Autodesk Inventor part; units mm, degrees
(part 4 of 4)
sketch "Sketch8" plane through (0, 0, 5) normal (0, 0, 1) x (1, 0, 0)
  line L0 (14.5144, 16.8863) -> (85.9619, 16.8863) construction
  line L1 (85.9619, 16.8863) -> (85.9619, -28.4978) construction
  line L2 (85.9619, -28.4978) -> (14.5144, -28.4978) construction
  line L3 (14.5144, -28.4978) -> (14.5144, 16.8863) construction
  line L4 (50.2381, 55.1961) -> (50.2381, 17.6773) construction
  line L5 (0, -39.5) -> (0, 79.5) construction
  spline S0 degree 2 poles (33.201, 11.0366) (32.522, 10.6859) (31.5146, 10.6859) knots 0 0 0 1 1 1
  spline S1 degree 2 poles (31.5146, 10.6859) (30.2066, 10.6859) (28.637, 12.3334) (28.637, 13.6748) knots 0 0 0 1 2 2 2
  spline S2 degree 2 poles (28.637, 13.6748) (28.637, 15.1108) (30.407, 16.8863) (31.7595, 16.8863) knots 0 0 0 1 2 2 2
  spline S3 degree 2 poles (31.7595, 16.8863) (32.6277, 16.8863) (33.201, 16.6414) knots 0 0 0 1 1 1
  line L6 (33.201, 16.6414) -> (33.201, 15.6507)
  spline S4 degree 2 poles (33.201, 15.6507) (32.5943, 16.0125) (31.8597, 16.0125) knots 0 0 0 1 1 1
  spline S5 degree 2 poles (31.8597, 16.0125) (30.8856, 16.0125) (29.6778, 14.7657) (29.6778, 13.7249) knots 0 0 0 1 2 2 2
  spline S6 degree 2 poles (29.6778, 13.7249) (29.6778, 12.7286) (30.8077, 11.5542) (31.7261, 11.5542) knots 0 0 0 1 2 2 2
  spline S7 degree 2 poles (31.7261, 11.5542) (32.5776, 11.5542) (33.201, 11.955) knots 0 0 0 1 1 1
  line L7 (33.201, 11.955) -> (33.201, 11.0366)
  line L8 (39.1565, 10.7861) -> (38.1602, 10.7861)
  line L9 (38.1602, 10.7861) -> (38.1602, 13.391)
  line L10 (38.1602, 13.391) -> (35.3327, 13.391)
  line L11 (35.3327, 13.391) -> (35.3327, 10.7861)
  line L12 (35.3327, 10.7861) -> (34.3365, 10.7861)
  line L13 (34.3365, 10.7861) -> (34.3365, 16.7861)
  line L14 (34.3365, 16.7861) -> (35.3327, 16.7861)
  line L15 (35.3327, 16.7861) -> (35.3327, 14.2648)
  line L16 (35.3327, 14.2648) -> (38.1602, 14.2648)
  line L17 (38.1602, 14.2648) -> (38.1602, 16.7861)
  line L18 (38.1602, 16.7861) -> (39.1565, 16.7861)
  line L19 (39.1565, 16.7861) -> (39.1565, 10.7861)
  line L20 (45.5684, 10.7861) -> (44.4775, 10.7861)
  line L21 (44.4775, 10.7861) -> (43.9376, 12.3112)
  line L22 (43.9376, 12.3112) -> (41.5776, 12.3112)
  line L23 (41.5776, 12.3112) -> (41.0545, 10.7861)
  line L24 (41.0545, 10.7861) -> (39.9691, 10.7861)
  line L25 (39.9691, 10.7861) -> (42.2177, 16.7861)
  line L26 (42.2177, 16.7861) -> (43.3365, 16.7861)
  line L27 (43.3365, 16.7861) -> (45.5684, 10.7861)
  line L28 (43.6704, 13.1238) -> (42.8411, 15.5171)
  spline S8 degree 2 poles (42.8411, 15.5171) (42.8021, 15.634) (42.7576, 15.8956) knots 0 0 0 1 1 1
  line L29 (42.7576, 15.8956) -> (42.7409, 15.8956)
  spline S9 degree 2 poles (42.7409, 15.8956) (42.7075, 15.6563) (42.6574, 15.5171) knots 0 0 0 1 1 1
  line L30 (42.6574, 15.5171) -> (41.8337, 13.1238)
  line L31 (41.8337, 13.1238) -> (43.6704, 13.1238)
  line L32 (49.7149, 10.7861) -> (46.3921, 10.7861)
  line L33 (46.3921, 10.7861) -> (46.3921, 16.7861)
  line L34 (46.3921, 16.7861) -> (47.3884, 16.7861)
  line L35 (47.3884, 16.7861) -> (47.3884, 11.6266)
  line L36 (47.3884, 11.6266) -> (49.7149, 11.6266)
  line L37 (49.7149, 11.6266) -> (49.7149, 10.7861)
  line L38 (57.0285, 10.7861) -> (56.0433, 10.7861)
  line L39 (56.0433, 10.7861) -> (56.0433, 14.6711)
  spline S10 degree 2 poles (56.0433, 14.6711) (56.0433, 15.1442) (56.099, 15.8344) knots 0 0 0 1 1 1
  line L40 (56.099, 15.8344) -> (56.0823, 15.8344)
  spline S11 degree 2 poles (56.0823, 15.8344) (55.9932, 15.4448) (55.9209, 15.2722) knots 0 0 0 1 1 1
  line L41 (55.9209, 15.2722) -> (54.1287, 10.7861)
  line L42 (54.1287, 10.7861) -> (53.4441, 10.7861)
  line L43 (53.4441, 10.7861) -> (51.6463, 15.2388)
  spline S12 degree 2 poles (51.6463, 15.2388) (51.5739, 15.4336) (51.4904, 15.8344) knots 0 0 0 1 1 1
  line L44 (51.4904, 15.8344) -> (51.4738, 15.8344)
  spline S13 degree 2 poles (51.4738, 15.8344) (51.5071, 15.4782) (51.5071, 14.66) knots 0 0 0 1 1 1
  line L45 (51.5071, 14.66) -> (51.5071, 10.7861)
  line L46 (51.5071, 10.7861) -> (50.5832, 10.7861)
  line L47 (50.5832, 10.7861) -> (50.5832, 16.7861)
  line L48 (50.5832, 16.7861) -> (51.9858, 16.7861)
  line L49 (51.9858, 16.7861) -> (53.561, 12.7898)
  spline S14 degree 2 poles (53.561, 12.7898) (53.7446, 12.3279) (53.8003, 12.1052) knots 0 0 0 1 1 1
  line L50 (53.8003, 12.1052) -> (53.817, 12.1052)
  spline S15 degree 2 poles (53.817, 12.1052) (53.9728, 12.5783) (54.0674, 12.8065) knots 0 0 0 1 1 1
  line L51 (54.0674, 12.8065) -> (55.676, 16.7861)
  line L52 (55.676, 16.7861) -> (57.0285, 16.7861)
  line L53 (57.0285, 16.7861) -> (57.0285, 10.7861)
  line L54 (61.8708, 10.7861) -> (58.5034, 10.7861)
  line L55 (58.5034, 10.7861) -> (58.5034, 16.7861)
  line L56 (58.5034, 16.7861) -> (61.7372, 16.7861)
  line L57 (61.7372, 16.7861) -> (61.7372, 15.9401)
  line L58 (61.7372, 15.9401) -> (59.4997, 15.9401)
  line L59 (59.4997, 15.9401) -> (59.4997, 14.2425)
  line L60 (59.4997, 14.2425) -> (61.5647, 14.2425)
  line L61 (61.5647, 14.2425) -> (61.5647, 13.4021)
  line L62 (61.5647, 13.4021) -> (59.4997, 13.4021)
  line L63 (59.4997, 13.4021) -> (59.4997, 11.6266)
  line L64 (59.4997, 11.6266) -> (61.8708, 11.6266)
  line L65 (61.8708, 11.6266) -> (61.8708, 10.7861)
  line L66 (67.5758, 10.7861) -> (66.4125, 10.7861)
  line L67 (66.4125, 10.7861) -> (65.4552, 12.3947)
  spline S16 degree 2 poles (65.4552, 12.3947) (65.3272, 12.6173) (65.0767, 12.929) (64.8207, 13.1294) (64.5201, 13.224) (64.3365, 13.224) knots 0 0 0 1 2 3 4 4 4
  line L68 (64.3365, 13.224) -> (63.9302, 13.224)
  line L69 (63.9302, 13.224) -> (63.9302, 10.7861)
  line L70 (63.9302, 10.7861) -> (62.9394, 10.7861)
  line L71 (62.9394, 10.7861) -> (62.9394, 16.7861)
  line L72 (62.9394, 16.7861) -> (64.9153, 16.7861)
  spline S17 degree 2 poles (64.9153, 16.7861) (65.3383, 16.7861) (66.0507, 16.5858) (66.5795, 16.1795) (66.8745, 15.5728) (66.8745, 15.1665) knots 0 0 0 1 2 3 4 4 4
  spline S18 degree 2 poles (66.8745, 15.1665) (66.8745, 14.8492) (66.6853, 14.3205) (66.3402, 13.903) (65.8504, 13.6136) (65.5443, 13.5357) knots 0 0 0 1 2 3 4 4 4
  line L73 (65.5443, 13.5357) -> (65.5443, 13.519)
  spline S19 degree 2 poles (65.5443, 13.519) (65.7057, 13.4243) (65.9506, 13.2017) (66.1676, 12.9679) (66.3791, 12.673) (66.5127, 12.4726) knots 0 0 0 1 2 3 4 4 4
  line L74 (66.5127, 12.4726) -> (67.5758, 10.7861)
  line L75 (63.9302, 15.9791) -> (63.9302, 14.031)
  line L76 (63.9302, 14.031) -> (64.7595, 14.031)
  spline S20 degree 2 poles (64.7595, 14.031) (64.9932, 14.031) (65.3773, 14.1757) (65.6667, 14.4429) (65.8225, 14.8269) (65.8225, 15.0663) knots 0 0 0 1 2 3 4 4 4
  spline S21 degree 2 poles (65.8225, 15.0663) (65.8225, 15.4948) (65.2771, 15.9791) (64.7706, 15.9791) knots 0 0 0 1 2 2 2
  line L77 (64.7706, 15.9791) -> (63.9302, 15.9791)
  line L78 (67.9988, 11.0255) -> (67.9988, 12.0496)
  spline S22 degree 2 poles (67.9988, 12.0496) (68.1379, 11.9216) (68.522, 11.7212) (68.945, 11.5876) (69.3736, 11.5097) (69.5517, 11.5097) knots 0 0 0 1 2 3 4 4 4
  spline S23 degree 2 poles (69.5517, 11.5097) (70.1806, 11.5097) (70.7984, 11.9271) (70.7984, 12.3279) knots 0 0 0 1 2 2 2
  spline S24 degree 2 poles (70.7984, 12.3279) (70.7984, 12.5394) (70.5925, 12.8511) (70.2251, 13.1127) (69.7242, 13.352) (69.4404, 13.48) knots 0 0 0 1 2 3 4 4 4
  spline S25 degree 2 poles (69.4404, 13.48) (69.1342, 13.6414) (68.611, 13.9809) (68.2214, 14.3817) (67.9988, 14.8937) (67.9988, 15.2388) knots 0 0 0 1 2 3 4 4 4
  spline S26 degree 2 poles (67.9988, 15.2388) (67.9988, 15.6618) (68.3773, 16.2852) (69.0007, 16.6915) (69.7966, 16.8863) (70.214, 16.8863) knots 0 0 0 1 2 3 4 4 4
  spline S27 degree 2 poles (70.214, 16.8863) (71.1546, 16.8863) (71.5832, 16.6748) knots 0 0 0 1 1 1
  line L79 (71.5832, 16.6748) -> (71.5832, 15.6897)
  spline S28 degree 2 poles (71.5832, 15.6897) (71.0712, 16.057) (70.2697, 16.057) knots 0 0 0 1 1 1
  spline S29 degree 2 poles (70.2697, 16.057) (70.047, 16.057) (69.6073, 15.9735) (69.2623, 15.7787) (69.0452, 15.4782) (69.0452, 15.2666) knots 0 0 0 1 2 3 4 4 4
  spline S30 degree 2 poles (69.0452, 15.2666) (69.0452, 15.0663) (69.2122, 14.7713) (69.535, 14.532) (69.9969, 14.2982) (70.3031, 14.1646) knots 0 0 0 1 2 3 4 4 4
  spline S31 degree 2 poles (70.3031, 14.1646) (70.6148, 14.0032) (71.1713, 13.6414) (71.5943, 13.2073) (71.8448, 12.6785) (71.8448, 12.339) knots 0 0 0 1 2 3 4 4 4
  spline S32 degree 2 poles (71.8448, 12.339) (71.8448, 11.8826) (71.4775, 11.2537) (70.8541, 10.8641) (70.0415, 10.6859) (69.5851, 10.6859) knots 0 0 0 1 2 3 4 4 4
  spline S33 degree 2 poles (69.5851, 10.6859) (69.4348, 10.6859) (68.9951, 10.7305) (68.5387, 10.8195) (68.1268, 10.9475) (67.9988, 11.0255) knots 0 0 0 1 2 3 4 4 4
  line L80 (32.5693, 5.2738) -> (30.4153, -0.7262)
  line L81 (30.4153, -0.7262) -> (29.3021, -0.7262)
  line L82 (29.3021, -0.7262) -> (27.1871, 5.2738)
  line L83 (27.1871, 5.2738) -> (28.2725, 5.2738)
  line L84 (28.2725, 5.2738) -> (29.753, 0.7209)
  spline S34 degree 2 poles (29.753, 0.7209) (29.8253, 0.5039) (29.8643, 0.2145) knots 0 0 0 1 1 1
  line L85 (29.8643, 0.2145) -> (29.881, 0.2145)
  spline S35 degree 2 poles (29.881, 0.2145) (29.9088, 0.4538) (30.0034, 0.7321) knots 0 0 0 1 1 1
  line L86 (30.0034, 0.7321) -> (31.5173, 5.2738)
  line L87 (31.5173, 5.2738) -> (32.5693, 5.2738)
  line L88 (36.7326, -0.7262) -> (33.3652, -0.7262)
  line L89 (33.3652, -0.7262) -> (33.3652, 5.2738)
  line L90 (33.3652, 5.2738) -> (36.599, 5.2738)
  line L91 (36.599, 5.2738) -> (36.599, 4.4278)
  line L92 (36.599, 4.4278) -> (34.3615, 4.4278)
  line L93 (34.3615, 4.4278) -> (34.3615, 2.7302)
  line L94 (34.3615, 2.7302) -> (36.4264, 2.7302)
  line L95 (36.4264, 2.7302) -> (36.4264, 1.8898)
  line L96 (36.4264, 1.8898) -> (34.3615, 1.8898)
  line L97 (34.3615, 1.8898) -> (34.3615, 0.1143)
  line L98 (34.3615, 0.1143) -> (36.7326, 0.1143)
  line L99 (36.7326, 0.1143) -> (36.7326, -0.7262)
  line L100 (42.4376, -0.7262) -> (41.2743, -0.7262)
  line L101 (41.2743, -0.7262) -> (40.317, 0.8824)
  spline S36 degree 2 poles (40.317, 0.8824) (40.189, 1.105) (39.9385, 1.4167) (39.6825, 1.6171) (39.3819, 1.7117) (39.1982, 1.7117) knots 0 0 0 1 2 3 4 4 4
  line L102 (39.1982, 1.7117) -> (38.7919, 1.7117)
  line L103 (38.7919, 1.7117) -> (38.7919, -0.7262)
  line L104 (38.7919, -0.7262) -> (37.8012, -0.7262)
  line L105 (37.8012, -0.7262) -> (37.8012, 5.2738)
  line L106 (37.8012, 5.2738) -> (39.7771, 5.2738)
  spline S37 degree 2 poles (39.7771, 5.2738) (40.2001, 5.2738) (40.9125, 5.0735) (41.4413, 4.6671) (41.7363, 4.0605) (41.7363, 3.6542) knots 0 0 0 1 2 3 4 4 4
  spline S38 degree 2 poles (41.7363, 3.6542) (41.7363, 3.3369) (41.547, 2.8081) (41.202, 2.3907) (40.7122, 2.1013) (40.406, 2.0234) knots 0 0 0 1 2 3 4 4 4
  line L107 (40.406, 2.0234) -> (40.406, 2.0067)
  spline S39 degree 2 poles (40.406, 2.0067) (40.5674, 1.912) (40.8123, 1.6894) (41.0294, 1.4556) (41.2409, 1.1607) (41.3745, 0.9603) knots 0 0 0 1 2 3 4 4 4
  line L108 (41.3745, 0.9603) -> (42.4376, -0.7262)
  line L109 (38.7919, 4.4668) -> (38.7919, 2.5187)
  line L110 (38.7919, 2.5187) -> (39.6212, 2.5187)
  spline S40 degree 2 poles (39.6212, 2.5187) (39.855, 2.5187) (40.2391, 2.6634) (40.5285, 2.9306) (40.6843, 3.3146) (40.6843, 3.554) knots 0 0 0 1 2 3 4 4 4
  spline S41 degree 2 poles (40.6843, 3.554) (40.6843, 3.9825) (40.1389, 4.4668) (39.6324, 4.4668) knots 0 0 0 1 2 2 2
  line L111 (39.6324, 4.4668) -> (38.7919, 4.4668)
  line L112 (48.0702, -0.7262) -> (46.9793, -0.7262)
  line L113 (46.9793, -0.7262) -> (46.4394, 0.7989)
  line L114 (46.4394, 0.7989) -> (44.0795, 0.7989)
  line L115 (44.0795, 0.7989) -> (43.5563, -0.7262)
  line L116 (43.5563, -0.7262) -> (42.471, -0.7262)
  line L117 (42.471, -0.7262) -> (44.7196, 5.2738)
  line L118 (44.7196, 5.2738) -> (45.8383, 5.2738)
  line L119 (45.8383, 5.2738) -> (48.0702, -0.7262)
  line L120 (46.1723, 1.6115) -> (45.343, 4.0048)
  spline S42 degree 2 poles (45.343, 4.0048) (45.304, 4.1217) (45.2595, 4.3833) knots 0 0 0 1 1 1
  line L121 (45.2595, 4.3833) -> (45.2428, 4.3833)
  spline S43 degree 2 poles (45.2428, 4.3833) (45.2094, 4.144) (45.1593, 4.0048) knots 0 0 0 1 1 1
  line L122 (45.1593, 4.0048) -> (44.3355, 1.6115)
  line L123 (44.3355, 1.6115) -> (46.1723, 1.6115)
  line L124 (55.0999, 4.4278) -> (53.3745, 4.4278)
  line L125 (53.3745, 4.4278) -> (53.3745, -0.7262)
  line L126 (53.3745, -0.7262) -> (52.3782, -0.7262)
  line L127 (52.3782, -0.7262) -> (52.3782, 4.4278)
  line L128 (52.3782, 4.4278) -> (50.6584, 4.4278)
  line L129 (50.6584, 4.4278) -> (50.6584, 5.2738)
  line L130 (50.6584, 5.2738) -> (55.0999, 5.2738)
  line L131 (55.0999, 5.2738) -> (55.0999, 4.4278)
  line L132 (59.3467, -0.7262) -> (55.9793, -0.7262)
  line L133 (55.9793, -0.7262) -> (55.9793, 5.2738)
  line L134 (55.9793, 5.2738) -> (59.2131, 5.2738)
  line L135 (59.2131, 5.2738) -> (59.2131, 4.4278)
  line L136 (59.2131, 4.4278) -> (56.9756, 4.4278)
  line L137 (56.9756, 4.4278) -> (56.9756, 2.7302)
  line L138 (56.9756, 2.7302) -> (59.0405, 2.7302)
  line L139 (59.0405, 2.7302) -> (59.0405, 1.8898)
  line L140 (59.0405, 1.8898) -> (56.9756, 1.8898)
  line L141 (56.9756, 1.8898) -> (56.9756, 0.1143)
  line L142 (56.9756, 0.1143) -> (59.3467, 0.1143)
  line L143 (59.3467, 0.1143) -> (59.3467, -0.7262)
  line L144 (65.3467, -0.7262) -> (64.2558, -0.7262)
  line L145 (64.2558, -0.7262) -> (63.7159, 0.7989)
  line L146 (63.7159, 0.7989) -> (61.3559, 0.7989)
  line L147 (61.3559, 0.7989) -> (60.8327, -0.7262)
  line L148 (60.8327, -0.7262) -> (59.7474, -0.7262)
  line L149 (59.7474, -0.7262) -> (61.996, 5.2738)
  line L150 (61.996, 5.2738) -> (63.1148, 5.2738)
  line L151 (63.1148, 5.2738) -> (65.3467, -0.7262)
  line L152 (63.4487, 1.6115) -> (62.6194, 4.0048)
  spline S44 degree 2 poles (62.6194, 4.0048) (62.5804, 4.1217) (62.5359, 4.3833) knots 0 0 0 1 1 1
  line L153 (62.5359, 4.3833) -> (62.5192, 4.3833)
  spline S45 degree 2 poles (62.5192, 4.3833) (62.4858, 4.144) (62.4357, 4.0048) knots 0 0 0 1 1 1
  line L154 (62.4357, 4.0048) -> (61.612, 1.6115)
  line L155 (61.612, 1.6115) -> (63.4487, 1.6115)
  line L156 (72.6157, -0.7262) -> (71.6305, -0.7262)
  line L157 (71.6305, -0.7262) -> (71.6305, 3.1588)
  spline S46 degree 2 poles (71.6305, 3.1588) (71.6305, 3.6319) (71.6862, 4.3221) knots 0 0 0 1 1 1
  line L158 (71.6862, 4.3221) -> (71.6695, 4.3221)
  spline S47 degree 2 poles (71.6695, 4.3221) (71.5804, 3.9325) (71.5081, 3.7599) knots 0 0 0 1 1 1
  line L159 (71.5081, 3.7599) -> (69.7159, -0.7262)
  line L160 (69.7159, -0.7262) -> (69.0313, -0.7262)
  line L161 (69.0313, -0.7262) -> (67.2335, 3.7265)
  spline S48 degree 2 poles (67.2335, 3.7265) (67.1611, 3.9213) (67.0776, 4.3221) knots 0 0 0 1 1 1
  line L162 (67.0776, 4.3221) -> (67.061, 4.3221)
  spline S49 degree 2 poles (67.061, 4.3221) (67.0943, 3.9658) (67.0943, 3.1477) knots 0 0 0 1 1 1
  line L163 (67.0943, 3.1477) -> (67.0943, -0.7262)
  line L164 (67.0943, -0.7262) -> (66.1704, -0.7262)
  line L165 (66.1704, -0.7262) -> (66.1704, 5.2738)
  line L166 (66.1704, 5.2738) -> (67.573, 5.2738)
  line L167 (67.573, 5.2738) -> (69.1481, 1.2775)
  spline S50 degree 2 poles (69.1481, 1.2775) (69.3318, 0.8156) (69.3875, 0.5929) knots 0 0 0 1 1 1
  line L168 (69.3875, 0.5929) -> (69.4042, 0.5929)
  spline S51 degree 2 poles (69.4042, 0.5929) (69.56, 1.066) (69.6546, 1.2942) knots 0 0 0 1 1 1
  line L169 (69.6546, 1.2942) -> (71.2632, 5.2738)
  line L170 (71.2632, 5.2738) -> (72.6157, 5.2738)
  line L171 (72.6157, 5.2738) -> (72.6157, -0.7262)
  point P0 (0, 0)
  constraints: 2 end point, 1 vertical, 3 other
sketch "Sketch9" plane through (0, 0, 0) normal (1, 0, 0) x (0, 1, 0)
  line L0 (49.5, 5) -> (22.5, 5)
  line L1 (22.5, 5) -> (39.4411, 29.6041)
  arc A0 (57.2132, 23.8426) -> (49.5, 5) centre (49.5, 16) ccw
  line L2 (62.5, 5) -> (25.2319, 5) projected
  line L3 (60.5, 5) -> (60.5, 28.4158) construction
  line L4 (39.4411, 29.6041) -> (44.6892, 37.2262) construction
  line L5 (44.6892, 37.2262) -> (59.5042, 28.4158) construction
  spline S0 degree 2 poles (39.4411, 29.6041) (44.6892, 37.2262) (59.5042, 28.4158) knots 1 1 1 2 2 2
  line L6 (59.5042, 28.4158) -> (57.2132, 23.8426)
  point P0 (0, 0)
  point P1 (17.5, 5)
  dimension "d57" = 5
  dimension "d58" = 2
  dimension "d59" = 22
  dimension "d60" = 16
  constraints: 8 end point, 2 point on circle, 2 point on line, 2 tangent, 1 centre point, 1 collinear, 1 horizontal, 1 vertical, 4 other
  measures "d57" distance of point (17.5, 5) L0.end
  measures "d58" distance of L3.start L2.start
  measures "d59" diameter of A0
  measures "d60" distance from line of L1 A0.centre
extrude "Extrusion8" add sketch "Sketch9" along normal blind 10 and the other way blind 10 separate body
chamfer "Chamfer2" distance 1 angle 45 3 edges at (0, 57.2132, 23.8426) (5, 59.5042, 28.4158) (-5, 59.5042, 28.4158)
fillet "Fillet3" radius 1 6 edges at (10, 39.141, 19.7002) (-10, 39.141, 19.7002) (10, 46.7878, 33.132) (10, 30.9705, 17.3021) (-10, 30.9705, 17.3021) (-10, 46.7878, 33.132)
extrude "Extrusion6" cut sketch "Sketch8" against normal blind 1 bodies 1
sketch "Sketch10" plane through (-9, 22.5, 5) normal (0, -0.8236391, 0.5671142) x (1, 0, 0)
  line L0 (5, 13.8121) -> (13, 13.8121)
  line L1 (13, 13.8121) -> (13, 16.8121)
  line L2 (13, 16.8121) -> (5, 16.8121)
  line L3 (5, 16.8121) -> (5, 13.8121)
  line L4 (0, 15.3121) -> (18, 15.3121) projected
  line L5 (5, 13.8121) -> (13, 16.8121) construction
  line L6 (13, 13.8121) -> (5, 16.8121) construction
  point P0 (9, -16.8783)
  point P1 (9, 15.3121)
  dimension "d69" = 3
  dimension "d70" = 8
  constraints: 12 end point, 3 midpoint, 2 parallel, 1 horizontal, 1 perpendicular
  measures "d69" distance of L0.end L1.end
  measures "d70" distance of L1.end L2.end
extrude "Extrusion9" cut sketch "Sketch10" against normal up to surface round surface about axis through (0, 49.5, 16) along (1, 0, 0) radius 11 far side no bodies 2
equation "\"d5\" = mountingScrewSize"
equation "\"d6\" = d5"
equation "\"d18\" = d6"
equation "\"d21\" = d20"
equation "\"d22\" = d20"
equation "\"d23\" = d20"
equation "\"d36\" = mountingScrewSize"
equation "\"mountingScrewSize\" = 3"
body "Solid1"
body "Solid2"
body "Solid3"
